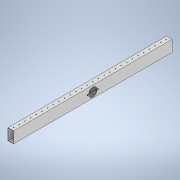
# Autodesk Inventor part: VerseFrame 28in
Saved by Autodesk Inventor 2020 (Build 240168000, 168)
## iProperties
Created: 2020-01-14
Part Number: VerseFrame 28in
Material: Generic
Document SubType Name: Modeling
Designer: aidan
Density: 1 g/cm^3
Appearance: Default
Author: aidan
Autodesk Inventor part; units mm, degrees
ref_plane "YZ Plane" through (0, 0, 0) normal (1, 0, 0) x (0, 1, 0)
ref_plane "XZ Plane" through (0, 0, 0) normal (0, 1, 0) x (-1, 0, 0)
ref_plane "XY Plane" through (0, 0, 0) normal (0, 0, 1) x (1, 0, 0)
sketch "Sketch1" plane through (0, 0, 0) normal (0, 0, 1) x (1, 0, 0)
  line L0 (-12.1708, 16.0073) -> (13.2292, 16.0073)
  line L1 (13.2292, 16.0073) -> (13.2292, -34.7927)
  line L2 (13.2292, -34.7927) -> (-12.1708, -34.7927)
  line L3 (-12.1708, -34.7927) -> (-12.1708, 16.0073)
  line L4 (11.9592, 14.7373) -> (-10.9008, 14.7373)
  line L5 (-10.9008, 14.7373) -> (-10.9008, -33.5227)
  line L6 (-10.9008, -33.5227) -> (11.9592, -33.5227)
  line L7 (11.9592, -33.5227) -> (11.9592, 14.7373)
  point P0 (0, 0)
  dimension "d0" = 25.4
  dimension "d1" = 50.8
  dimension "d2" = 1.27
  constraints: 16 end point, 4 parallel, 2 perpendicular, 1 horizontal, 3 other
  measures "d0" distance of L0.start L0.end
  measures "d1" distance of L0.end L1.end
  measures "d2" distance between parallel lines of L0 L4
extrude "Extrusion1" add sketch "Sketch1" along normal blind 762
sketch "Sketch2" plane through (-12.1708, 16.0073, 0) normal (0, 1, 0) x (1, 0, 0)
  circle A0 centre (12.7, -12.7) radius 1.7272
  line L0 (25.4, 0) -> (0, 0) projected
  line L1 (0, 0) -> (0, -762) projected
  point P0 (12.1708, 0)
  dimension "d5" = 3.4544
  dimension "d6" = 12.7
  dimension "d7" = 12.7
  constraints: 1 centre point
  measures "d5" diameter of A0
  measures "d6" distance from line of L0 A0.centre
  measures "d7" distance from line of L1 A0.centre
extrude "Extrusion2" cut sketch "Sketch2" against normal through all
pattern_linear "Rectangular Pattern1" count 30 spacing 25.4 along (0, 0, 1) of "Extrusion2"
sketch "Sketch3" plane through (-12.1708, 16.0073, 0) normal (0, 1, 0) x (1, 0, 0)
  line L0 (0, 0) -> (25.4, 0)
  line L1 (25.4, 0) -> (25.4, -50.8)
  line L2 (25.4, -50.8) -> (0, -50.8)
  line L3 (0, -50.8) -> (0, 0)
  line L4 (25.4, 0) -> (0, 0) projected
  line L5 (0, 0) -> (0, -762) projected
  point P0 (12.1708, 0)
  dimension "d13" = 25.4
  dimension "d14" = 50.8
  constraints: 8 end point, 2 collinear, 2 parallel, 1 horizontal, 1 perpendicular
  measures "d13" distance of L1.end L2.end
  measures "d14" distance of L0.end L1.end
extrude "Extrusion3" cut sketch "Sketch3" against normal through all
sketch "Sketch4" plane through (13.2292, -34.7927, 762) normal (1, 0, 0) x (0, 0, -1)
  circle A0 centre (355.6, 23.8125) radius 19.05
  circle A1 centre (331.7875, 23.8125) radius 2.4892
  circle A2 centre (379.4125, 23.8125) radius 2.4892
  line L0 (211.1702, 23.8125) -> (474.5961, 23.8125) construction
  line L1 (711.2, 50.8) -> (0, 50.8) projected
  line L2 (355.6, 71.9333) -> (355.6, -75.2373) construction
  line L3 (0, 0) -> (0, 50.8) projected
  point P0 (762, 34.7927)
  dimension "d17" = 38.1
  dimension "d18" = 26.9875
  dimension "d19" = 47.625
  dimension "d20" = 4.9784
  dimension "d21" = 355.6
  dimension "d22" = 23.8125
  constraints: 4 end point, 4 point on line, 3 centre point, 1 equal radius, 1 horizontal, 1 vertical
  measures "d17" diameter of A0
  measures "d18" distance between parallel lines of L1 L0
  measures "d19" distance of A2.centre A1.centre
  measures "d20" diameter of A2
  measures "d21" distance between parallel lines of L2 L3
  measures "d22" distance from line of L2 A1.centre
extrude "Extrusion4" cut sketch "Sketch4" against normal blind 25.4
body "Solid1"
